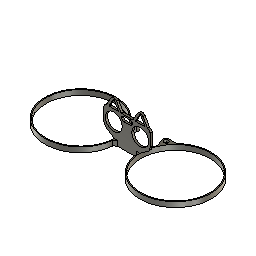
Prop Guard Front v35 (Autodesk Fusion 360 design; units mm, degrees)
Autodesk Fusion 360 part; units mm, degrees
note: some values were not read from the file. Chosen so that the rebuilt part matches the saved one: which face or edge a step refers to; which pieces of a blend or face edit are solid. Set by a fixed rule: which sketch regions a step uses.
sketch "Sketch1" plane through (0, 0, 0) normal (0, 0, 1) x (1, 0, 0)
  line L0 (25, 40) -> (-25, 40)
  line L1 (-25, 40) -> (-25, -40)
  line L2 (-25, -40) -> (25, -40)
  line L3 (25, -40) -> (25, 40)
  line L4 (25, 40) -> (-25, -40) construction
  line L5 (-25, 40) -> (25, -40) construction
  line L6 (25, 40) -> (46.6506, 52.5)
  line L7 (25, 40) -> (55, 40) construction
  line L8 (0, 40) -> (0, -40)
  line L9 (-25, 0) -> (25, 0)
  line L10 (25, 40) -> (23.5, 42.5981)
  line L11 (23.5, 42.5981) -> (45.1506, 55.0981)
  line L12 (45.1506, 55.0981) -> (46.6506, 52.5)
  line L13 (25, 40) -> (26.5, 37.4019)
  line L14 (26.5, 37.4019) -> (48.1506, 49.9019)
  line L15 (23.5, 42.5981) -> (19, 40)
  line L16 (26.5, 37.4019) -> (25, 36.5359)
  line L17 (48.1506, 49.9019) -> (46.6506, 52.5)
  circle A0 centre (46.6506, 52.5) radius 12
  circle A1 centre (46.6506, 52.5) radius 10
  line L18 (46.6506, 52.5) -> (41.6506, 61.1603)
  line L19 (46.6506, 52.5) -> (55.3109, 57.5)
  line L20 (46.6506, 52.5) -> (51.6506, 43.8397)
  circle A2 centre (46.6506, 52.5) radius 1.5
  line L21 (46.6506, 52.5) -> (51.8468, 55.5)
  line L22 (46.6506, 52.5) -> (43.6506, 57.6962)
  circle A3 centre (-46.6506, 52.5) radius 1.5
  line L23 (-23.5, 42.5981) -> (-45.1506, 55.0981)
  line L24 (-26.5, 37.4019) -> (-48.1506, 49.9019)
  circle A4 centre (-46.6506, 52.5) radius 12
  circle A5 centre (-46.6506, 52.5) radius 10
  line L25 (-26.5, 37.4019) -> (-25, 36.5359)
  line L26 (-23.5, 42.5981) -> (-19, 40)
  circle A6 centre (-46.6506, -52.5) radius 10
  line L27 (-26.5, -37.4019) -> (-48.1506, -49.9019)
  line L28 (-23.5, -42.5981) -> (-45.1506, -55.0981)
  line L29 (-23.5, -42.5981) -> (-19, -40)
  line L30 (-26.5, -37.4019) -> (-25, -36.5359)
  line L31 (23.5, -42.5981) -> (19, -40)
  line L32 (26.5, -37.4019) -> (25, -36.5359)
  line L33 (26.5, -37.4019) -> (48.1506, -49.9019)
  line L34 (23.5, -42.5981) -> (45.1506, -55.0981)
  circle A7 centre (46.6506, -52.5) radius 12
  circle A8 centre (46.6506, -52.5) radius 10
  circle A9 centre (46.6506, -52.5) radius 1.5
  circle A10 centre (-46.6506, -52.5) radius 10
  circle A11 centre (-46.6506, -52.5) radius 12
  line L35 (25, 0) -> (25, -40)
  line L36 (0, 0) -> (0, -9)
  line L37 (0, -9) -> (0, -10.6)
  line L38 (0, -9) -> (0, -7.4)
  line L39 (0, -10.6) -> (14, -10.6)
  line L40 (0, -9) -> (1, -9)
  line L41 (0, -7.4) -> (14, -7.4)
  line L42 (14, -10.6) -> (14, -7.4)
  line L43 (-14, -10.6) -> (-14, -7.4)
  line L44 (0, -7.4) -> (-14, -7.4)
  line L45 (0, -10.6) -> (-14, -10.6)
  line L46 (0, 7.4) -> (-14, 7.4)
  line L47 (-14, 10.6) -> (-14, 7.4)
  line L48 (0, 10.6) -> (-14, 10.6)
  line L49 (0, 10.6) -> (14, 10.6)
  line L50 (0, 7.4) -> (14, 7.4)
  line L51 (14, 10.6) -> (14, 7.4)
  line L52 (19, -40) -> (25.9282, -44)
  line L53 (25, -36.5359) -> (25, -31.5359)
  line L54 (19, -40) -> (16, -40)
  line L55 (14.6699, -37.5) -> (34.8771, -37.5) construction
  circle A12 centre (46.6506, -52.5) radius 35
  circle A13 centre (46.6506, -52.5) radius 34
  circle A14 centre (-46.6506, -52.5) radius 35
  circle A15 centre (-46.6506, -52.5) radius 34
  circle A16 centre (-46.6506, 52.5) radius 35
  circle A17 centre (-46.6506, 52.5) radius 34
  circle A18 centre (46.6506, 52.5) radius 35
  circle A19 centre (46.6506, 52.5) radius 34
  line L56 (46.6506, -52.5) -> (46.6506, 52.5)
  line L57 (46.6506, -52.5) -> (-46.6506, -52.5)
  line L58 (46.6506, -52.5) -> (46.6506, -53.5)
  line L59 (-46.6506, -52.5) -> (-46.6506, -53.5)
  line L60 (-46.6506, -53.5) -> (46.6506, -53.5)
  line L61 (46.6506, -52.5) -> (46.6506, -51.5)
  line L62 (-46.6506, -51.5) -> (46.6506, -51.5)
  line L63 (-46.6506, -52.5) -> (-46.6506, -51.5)
  line L64 (-46.6506, 53.5) -> (46.6506, 53.5)
  line L65 (-46.6506, 51.5) -> (46.6506, 51.5)
  line L66 (46.6506, 0) -> (47.1506, 0)
  line L67 (47.1506, 0) -> (47.1506, -17.5036)
  line L68 (47.1506, 0) -> (47.1506, 17.5036)
  line L69 (46.1506, 0) -> (46.1506, 17.5036)
  line L70 (46.1506, 0) -> (46.1506, -17.5036)
  line L71 (-46.1506, 0) -> (-46.1506, 17.5036)
  line L72 (-47.1506, 0) -> (-47.1506, 17.5036)
  line L73 (-47.1506, 0) -> (-47.1506, -17.5036)
  line L74 (-46.1506, 0) -> (-46.1506, -17.5036)
  line L75 (-47.1506, 0) -> (60, 0)
  line L76 (25, -40) -> (25, -30.5)
  line L77 (25, -30.5) -> (15.5, -30.5)
  circle A20 centre (15.5, -30.5) radius 1.3
  circle A21 centre (15.5, -30.5) radius 3.6
  circle A22 centre (-15.5, -30.5) radius 3.6
  circle A23 centre (-15.5, -30.5) radius 1.3
  line L78 (15.5, -30.5) -> (15.5, -29.2)
  circle A24 centre (15.5, -30.5) radius 2.2
  circle A25 centre (-15.5, -30.5) radius 2.2
  point P0 (-46.6506, -52.5)
  dimension "d1" = 50
  dimension "d2" = 80
  dimension "d4" = 25
  dimension "d5" = 30
  dimension "d6" = 3
  dimension "d7" = 25
  dimension "d8" = 24
  dimension "d9" = 20
  dimension "d10" = 3
  dimension "d11" = 6
  dimension "d13" = 6
  dimension "d23" = 9
  dimension "d24" = 1.6
  dimension "d25" = 1.6
  dimension "d26" = 14
  dimension "d51" = 8
  dimension "d76" = 5
  dimension "d77" = 3
  dimension "d88" = 5
  dimension "d130" = 70
  dimension "d131" = 68
  dimension "d132" = 1
  dimension "d133" = 0.5
  dimension "d140" = 9.5
  dimension "d141" = 9.5
  dimension "d142" = 2.6
  dimension "d143" = 7.2
  dimension "d147" = 4.4
  constraint horizontal L0
  constraint perpendicular L0 L1
  constraint parallel L0 L2
  constraint parallel L1 L3
  constraint coincident L4 L36.start
  constraint coincident L5 L36.start
  constraint coincident L36.start origin
  constraint horizontal L7
  constraint midpoint L0 L8.start
  constraint midpoint L2 L8.end
  constraint midpoint L1 L9.start
  constraint midpoint L3 L9.end
  constraint perpendicular L6 L10
  constraint perpendicular L10 L11
  constraint symmetric L0.start L6 L3.end
  constraint symmetric L6 L10.end L13.end
  constraint symmetric L6 L11.end L14.end
  constraint coincident L0 L15.end
  constraint perpendicular L10 L15
  constraint coincident L3 L16.end
  constraint perpendicular L13 L16
  constraint symmetric L12.end L6 L17.end
  constraint coincident L6.end L12.end
  constraint concentric A0 A1
  constraint coincident A1 L18.end
  constraint parallel L12 L18
  constraint coincident A1 L19.end
  constraint perpendicular L12 L19
  constraint coincident A1 L20.end
  constraint perpendicular L19 L20
  constraint perpendicular L20 L21
  constraint parallel L18 L22
  constraint symmetric L8 L10.end L23.start
  constraint symmetric L8 L11.end L23.end
  constraint symmetric L8 L13.end L24.start
  constraint symmetric L8 L14.end L24.end
  constraint symmetric L8 L15.end L26.end
  constraint symmetric L8 L16.end L25.end
  constraint symmetric L8 A0 A4
  constraint symmetric L8 A1 A5
  constraint symmetric L8 A2 A3
  constraint symmetric L9 L10.end L31.start
  constraint symmetric L9 L11.end L34.end
  constraint symmetric L9 L13.end L32.start
  constraint symmetric L9 L14.end L33.end
  constraint symmetric L9 L15.end L31.end
  constraint symmetric L9 L16.end L32.end
  constraint symmetric L9 A0 A7
  constraint symmetric L9 A1 A8
  constraint symmetric L9 A2 A9
  constraint symmetric L9 L23.start L28.start
  constraint symmetric L9 L23.end L28.end
  constraint symmetric L9 L24.start L27.start
  constraint symmetric L9 L24.end L27.end
  constraint symmetric L9 A3.centre P0
  constraint symmetric L9 A5 A6
  constraint symmetric L9 L25.end L30.end
  constraint symmetric L9 L26.end L29.end
  constraint symmetric L9 A5 A10
  constraint symmetric L9 A4 A11
  constraint perpendicular L9 L36
  constraint parallel L8 L37
  constraint parallel L36 L38
  constraint perpendicular L37 L39
  constraint perpendicular L38 L40
  constraint symmetric L37.end L40 L38.end
  constraint symmetric L39.end L40 L41.end
  constraint symmetric L8 L37.end L39.start
  constraint symmetric L8 L39.end L43.start
  constraint symmetric L8 L38.end L41.start
  constraint symmetric L8 L41.end L43.end
  constraint symmetric L9 L37.end L48.start
  constraint symmetric L9 L39.end L49.end
  constraint symmetric L9 L38.end L46.start
  constraint symmetric L9 L41.end L50.end
  constraint symmetric L9 L43.start L47.start
  constraint symmetric L9 L43.end L46.end
  constraint parallel L34 L52
  constraint parallel L2 L54
  constraint horizontal L55
  constraint concentric A8 A12
  constraint concentric A9 A13
  constraint symmetric L8 A12 A14
  constraint symmetric L8 A13 A15
  constraint symmetric L9 A12 A18
  constraint symmetric L9 A13 A19
  constraint symmetric L9 A14 A16
  constraint symmetric L9 A15 A17
  constraint coincident A7.centre A8.centre
  constraint coincident P0 A6.centre
  constraint perpendicular L57 L58
  constraint symmetric L8 A7.centre P0
  constraint symmetric L8 L58.end L59.end
  constraint symmetric L57 A7.centre A8.centre
  constraint symmetric L57 L58.end L61.end
  constraint symmetric L57 P0 A6.centre
  constraint symmetric L57 L59.end L62.start
  constraint symmetric L9 L58.end L64.end
  constraint symmetric L9 L59.end L64.start
  constraint symmetric L9 L61.end L65.end
  constraint symmetric L9 L62.start L65.start
  constraint midpoint L56 L66.start
  constraint perpendicular L56 L66
  constraint coincident A12 L67.end
  constraint perpendicular L66 L67
  constraint coincident A18 L68.end
  constraint perpendicular L66 L68
  constraint symmetric L56 L66.end L69.start
  constraint symmetric L56 L67.end L70.end
  constraint symmetric L56 L68.end L69.end
  constraint symmetric L8 L66.end L72.start
  constraint symmetric L8 L67.end L73.end
  constraint symmetric L8 L68.end L72.end
  constraint symmetric L8 L69.start L71.start
  constraint symmetric L8 L69.end L71.end
  constraint symmetric L8 L70.end L74.end
  constraint perpendicular L71 L75
  constraint perpendicular L2 L76
  constraint perpendicular L35 L77
  constraint coincident L77.end A20.centre
  constraint concentric A20 A21
  constraint symmetric L8 A20 A23
  constraint symmetric L8 A21 A22
  constraint coincident A20 L78.end
  constraint perpendicular L77 L78
  constraint concentric A20 A24
  constraint symmetric L8 A24 A25
  measures "d1" distance of L1.end L2.end
  measures "d2" distance of L0.end L1.end
  measures "d4" distance of L0.start L6.end
  measures "d5" angle of L6 L7
  measures "d6" distance of L0.start L10.end
  measures "d7" distance of L10.end L11.end
  measures "d8" diameter of A0
  measures "d9" diameter of A1
  measures "d10" diameter of A2
  measures "d11" distance of L6.end L21.end
  measures "d13" distance of L6.end L22.end
  measures "d23" distance of L36.start L36.end
  measures "d24" distance of L36.end L37.end
  measures "d25" distance of L36.end L38.end
  measures "d26" distance of L37.end L39.end
  measures "d51" distance of L31.end L52.end
  measures "d76" distance of L32.end L53.end
  measures "d77" distance of L31.end L54.end
  measures "d88" distance of L31.end L55.start
  measures "d130" diameter of A12
  measures "d131" diameter of A13
  measures "d132" distance of A7.centre L58.end
  measures "d133" distance of L66.start L66.end
  measures "d140" distance of L2.end L76.end
  measures "d141" distance of L76.end L77.end
  measures "d142" diameter of A20
  measures "d143" diameter of A21
  measures "d147" diameter of A24
extrude "Extrude6" add sketch "Sketch1" along normal blind 5 contours L3 L35 A12 A13 L56 | L3 L35 A12 A13 L77 | L2 A12 A13 L77 A21 | A12 A13 L56 L60 | A12 A21 | A12 A21 | L1 L2 A14 A15 A22 | L1 A14 A15 L60 | L2 A12 A13 L62 | A14 A22 | A14 A22 | A12 A13 L57 L60 | A12 A13 L57 L62 | L2 A14 A15 L62 | A14 A15 L57 L60 | A12 A14 L57 L60 | A12 A14 L57 L62 | A14 A15 L57 L62 | A24 | A25
chamfer "Chamfer39" distance 5 angle 45 4 edges at (17.1185, -33.7157, 2.5) (19.0718, -30.9499, 2.5) (-19.0718, -30.9499, 2.5) (-17.1185, -33.7157, 2.5)
chamfer "Chamfer40" distance 2 angle 45 4 edges at (11.6649, -51.5, 2.5) (11.6649, -53.5, 2.5) (-11.6649, -51.5, 2.5) (-11.6649, -53.5, 2.5)
extrude "Extrude7" cut sketch "Sketch1" along normal blind 5 and the other way blind -3 contours A24 | A25
sketch "Sketch3" plane through (0, 0, 5) normal (0, 0, 1) x (-1, 0, 0)
  circle A0 centre (-15.5, 30.5) radius 2.2
  circle A1 centre (15.5, 30.5) radius 2.2
  circle A2 centre (46.6506, 52.5) radius 34
  circle A3 centre (-46.6506, 52.5) radius 34
  arc A4 (12.3438, 32.2316) -> (16.0764, 26.9464) centre (15.5, 30.5) ccw
  line L0 (16.0764, 26.9464) -> (22.4239, 27.24)
  arc A5 (22.4239, 27.24) -> (11.7792, 55.4967) centre (46.6506, 52.5) ccw
  line L1 (11.7792, 55.4967) -> (9.6649, 53.5)
  line L2 (9.6649, 53.5) -> (-9.6649, 53.5)
  line L3 (-9.6649, 53.5) -> (-11.7792, 55.4967)
  arc A6 (-11.7792, 55.4967) -> (-22.4239, 27.24) centre (-46.6506, 52.5) ccw
  line L4 (-22.4239, 27.24) -> (-16.0764, 26.9464)
  arc A7 (-16.0764, 26.9464) -> (-12.3438, 32.2316) centre (-15.5, 30.5) ccw
  line L5 (-12.3438, 32.2316) -> (-14.7432, 38.1155)
  arc A8 (-14.7432, 38.1155) -> (-11.7792, 49.5033) centre (-46.6506, 52.5) ccw
  line L6 (-11.7792, 49.5033) -> (-9.6649, 51.5)
  line L7 (-9.6649, 51.5) -> (9.6649, 51.5)
  line L8 (9.6649, 51.5) -> (11.7792, 49.5033)
  arc A9 (11.7792, 49.5033) -> (14.7432, 38.1155) centre (46.6506, 52.5) ccw
  line L9 (14.7432, 38.1155) -> (12.3438, 32.2316)
  line L10 (11.7792, 49.5033) -> (12.783, 49.5033)
  line L11 (11.7792, 55.4967) -> (12.783, 55.4967)
  line L12 (-11.7792, 49.5033) -> (-12.783, 49.5033)
  line L13 (-11.7792, 55.4967) -> (-12.783, 55.4967)
  line L14 (9.6649, 51.5) -> (12.6653, 51.5)
  line L15 (9.6649, 53.5) -> (12.6653, 53.5)
  line L16 (-9.6649, 51.5) -> (-12.6653, 51.5)
  line L17 (-9.6649, 53.5) -> (-12.6653, 53.5)
  line L18 (12.6653, 51.5) -> (22.6653, 51.5)
  line L19 (0, 51.5) -> (0, 53.5)
  line L20 (0, 52.5) -> (12.6506, 52.5)
  line L21 (12.6653, 53.5) -> (22.6653, 53.5)
  line L22 (22.6653, 51.5) -> (22.6653, 53.5)
  line L23 (-12.6653, 51.5) -> (-22.6653, 51.5)
  line L24 (-22.6653, 51.5) -> (-22.6653, 53.5)
  line L25 (-12.6653, 53.5) -> (-22.6653, 53.5)
  dimension "d170" = 10
  constraint coincident L8.end A9.start
  constraint coincident A2 L10.end
  constraint horizontal L10
  constraint coincident A5.end L1.start
  constraint coincident A2 L11.end
  constraint parallel L10 L11
  constraint coincident A8.end L6.start
  constraint coincident A3 L12.end
  constraint parallel L11 L12
  constraint coincident L3.end A6.start
  constraint coincident A3 L13.end
  constraint parallel L7 L13
  constraint coincident L7.end L8.start
  constraint coincident A2 L14.end
  constraint parallel L7 L14
  constraint coincident L1.end L2.start
  constraint coincident A2 L15.end
  constraint parallel L2 L15
  constraint coincident L6.end L7.start
  constraint coincident A3 L16.end
  constraint parallel L7 L16
  constraint coincident L2.end L3.start
  constraint coincident A3 L17.end
  constraint parallel L2 L17
  constraint parallel L14 L18
  constraint midpoint L7 L19.start
  constraint midpoint L2 L19.end
  constraint midpoint L19 L20.start
  constraint coincident A2 L20.end
  constraint perpendicular L19 L20
  constraint symmetric L14.end L20 L15.end
  constraint symmetric L18.end L20 L21.end
  constraint symmetric L14.end L19 L16.end
  constraint symmetric L18.end L19 L23.end
  constraint symmetric L19 L15.end L17.end
  constraint symmetric L19 L21.end L24.end
  measures "d170" distance of L14.end L18.end
extrude "Extrude8" add sketch "Sketch3" along normal blind 35 contours A2 L18 L21 L22 | A2 L2 L15 L19 L20 | A2 L7 L14 L19 L20 | A3 L2 L7 L16 L17 L19 | A3 L23 L24 L25 picked at (19.3271, 52.5) picked at (-19.3271, 52.5)
sketch "Sketch5" plane through (0, -53.5, 0) normal (0, -1, 0) x (1, 0, 0)
  line L0 (-9.6649, 5) -> (-9.6649, 0)
  line L1 (-9.6649, 0) -> (9.6649, 0)
  line L2 (9.6649, 0) -> (9.6649, 5)
  line L3 (9.6649, 5) -> (12.6653, 5)
  line L4 (12.6653, 5) -> (22.6653, 5)
  line L5 (22.6653, 5) -> (22.6653, 40)
  line L6 (22.6653, 40) -> (-22.6653, 40)
  line L7 (-22.6653, 40) -> (-22.6653, 5)
  line L8 (-22.6653, 5) -> (-12.6653, 5)
  line L9 (-12.6653, 5) -> (-9.6649, 5)
  line L10 (0, 40) -> (0, 19)
  line L11 (0, 19) -> (-13, 19)
  circle A0 centre (-13, 19) radius 8.25
  circle A1 centre (13, 19) radius 8.25
  line L12 (0, 40) -> (0, 30)
  line L13 (0, 30) -> (-22.6653, 30)
  line L14 (-22.6653, 30) -> (-12.3126, 30) construction
  line L15 (22.6653, 30) -> (12.3126, 30) construction
  line L16 (0, 30) -> (22.6653, 30)
  line L17 (0, 40) -> (0, 28.5)
  line L18 (0, 28.5) -> (-5.2, 28.5)
  line L19 (-5.2, 28.5) -> (-5.2, 24)
  line L20 (0, 28.5) -> (5.2, 28.5)
  line L21 (5.2, 28.5) -> (5.2, 24)
  line L22 (5.2, 24) -> (-5.2, 24)
  line L23 (-22.6653, 30) -> (-12.0236, 30) construction
  line L24 (0, 19) -> (0, 10.5)
  line L25 (5.4, 12) -> (-5.4, 12)
  line L26 (-5.4, 12) -> (-5.4, 9)
  line L27 (-5.4, 9) -> (5.4, 9)
  line L28 (5.4, 9) -> (5.4, 12)
  line L29 (5.4, 12) -> (-5.4, 9) construction
  line L30 (-5.4, 12) -> (5.4, 9) construction
  line L31 (-13, 19) -> (-13, 40)
  line L32 (-13, 40) -> (-11.5, 40)
  line L33 (-11.5, 40) -> (-5.7265, 30)
  line L34 (-14.5, 40) -> (-20.2735, 30)
  line L35 (11.5, 40) -> (5.7265, 30)
  line L36 (14.5, 40) -> (20.2735, 30)
  line L37 (-13, 40) -> (-13, 38)
  line L38 (-17.3868, 35) -> (-15.6547, 34)
  line L39 (-15.6547, 34) -> (-17.9641, 30)
  line L40 (-13, 38) -> (-15.6547, 38)
  line L41 (-15.6547, 34) -> (-13.3453, 38)
  line L42 (-15.6547, 34) -> (-11.3, 34) construction
  line L43 (-10.3453, 34) -> (-12.6547, 38)
  line L44 (-13, 38) -> (-10.3453, 38)
  line L45 (-10.3453, 34) -> (-8.0359, 30)
  line L46 (10.3453, 34) -> (12.6547, 38)
  line L47 (15.6547, 34) -> (13.3453, 38)
  line L48 (13, 38) -> (10.3453, 38)
  line L49 (13, 38) -> (15.6547, 38)
  line L50 (10.3453, 34) -> (8.0359, 30)
  line L51 (15.6547, 34) -> (17.9641, 30)
  point P0 (0, 10.5)
  dimension "d171" = 21
  dimension "d172" = 13
  dimension "d173" = 16.5
  dimension "d176" = 10
  dimension "d189" = 11.5
  dimension "d190" = 5.2
  dimension "d191" = 4.5
  dimension "d213" = 8.5
  dimension "d230" = 10.8
  dimension "d231" = 3
  dimension "d232" = 1.5
  dimension "d233" = 120
  dimension "d240" = 2
  dimension "d241" = 2
  dimension "d242" = 90
  dimension "d243" = 60
  constraint midpoint L6 L10.start
  constraint perpendicular L6 L10
  constraint perpendicular L10 L11
  constraint coincident L11.end A0.centre
  constraint symmetric L10 A0 A1
  constraint perpendicular L6 L12
  constraint coincident L7 L13.end
  constraint perpendicular L7 L13
  constraint horizontal L14
  constraint symmetric L13.start L12 L16.start
  constraint symmetric L12 L13.end L15.start
  constraint symmetric L12 L14.end L15.end
  constraint perpendicular L6 L17
  constraint perpendicular L12 L18
  constraint perpendicular L18 L19
  constraint symmetric L12 L17.end L18.start
  constraint symmetric L12 L18.end L20.end
  constraint symmetric L12 L19.end L21.end
  constraint horizontal L23
  constraint perpendicular L11 L24
  constraint horizontal L25
  constraint perpendicular L25 L26
  constraint parallel L25 L27
  constraint parallel L26 L28
  constraint coincident L29 P0
  constraint coincident L30 P0
  constraint coincident P0 L24.end
  constraint coincident L6 L31.end
  constraint perpendicular L6 L31
  constraint perpendicular L31 L32
  constraint coincident L13 L33.end
  constraint symmetric L31 L32.end L34.start
  constraint symmetric L31 L33.end L34.end
  constraint symmetric L17 L32.end L35.start
  constraint symmetric L17 L33.end L35.end
  constraint symmetric L17 L34.start L36.start
  constraint symmetric L17 L34.end L36.end
  constraint coincident L31 L37.end
  constraint midpoint L34 L38.start
  constraint perpendicular L34 L38
  constraint coincident L14 L39.end
  constraint coincident L34 L40.end
  constraint perpendicular L37 L40
  constraint horizontal L42
  constraint coincident L40 L41.end
  constraint symmetric L31 L37.end L40.start
  constraint symmetric L31 L38.end L43.start
  constraint symmetric L31 L39.end L45.end
  constraint symmetric L31 L40.end L44.end
  constraint symmetric L31 L41.end L43.end
  constraint symmetric L12 L37.end L48.start
  constraint symmetric L12 L38.end L47.start
  constraint symmetric L12 L39.end L51.end
  constraint symmetric L12 L40.end L49.end
  constraint symmetric L12 L41.end L47.end
  constraint symmetric L12 L43.start L46.start
  constraint symmetric L12 L43.end L46.end
  constraint symmetric L12 L44.end L48.end
  constraint symmetric L12 L45.end L50.end
  measures "d171" distance of L10.start L10.end
  measures "d172" distance of L10.end L11.end
  measures "d173" diameter of A0
  measures "d176" distance of L10.start L12.end
  measures "d189" distance of L10.start L17.end
  measures "d190" distance of L17.end L18.end
  measures "d191" distance of L18.end L19.end
  measures "d213" distance of L10.end P0
  measures "d230" distance of L26.end L27.end
  measures "d231" distance of L25.end L26.end
  measures "d232" distance of L31.end L32.end
  measures "d233" angle of L32 L33
  measures "d240" distance of L31.end L37.end
  measures "d241" distance of L38.start L38.end
  measures "d242" angle of L38 L39
  measures "d243" angle of L41 L42
extrude "Extrude12" cut sketch "Sketch5" against normal blind 2 contours L6 L7 L13 L34 | L13 L31 L39 L40 L41 | L5 L6 L16 L36 | L13 L31 L43 L44 L45 | L6 L10 L12 L13 L17 L33 | L11 A0 L31 | L11 A0 L31 | L16 L46 L47 L48 L49 L50 L51 | L6 L10 L12 L16 L17 L35 | L10 L20 L21 L22 | L10 L18 L19 L22 | A1
fillet "Fillet7" radius 2 4 edges at (5.2, -52.5, 28.5) (5.2, -52.5, 24) (-5.2, -52.5, 24) (-5.2, -52.5, 28.5)
chamfer "Chamfer41" distance 7 distance2 10 1 edges at (-22.6653, -52.5, 5) measured on face at (-22.6653, -52.1667, 13.3333)
chamfer "Chamfer42" distance 10 distance2 7 1 edges at (22.6653, -52.5, 5) measured on face at (19.3277, -52.3889, 5)
fillet "Fillet17" radius 3.25 4 edges at (-11.5, -52.5, 40) (-14.5, -52.5, 40) (14.5, -52.5, 40) (11.5, -52.5, 40)
fillet "Fillet18" radius 0.5 8 edges at (-12.6547, -52.5, 38) (-13.3453, -52.5, 38) (13.3453, -52.5, 38) (12.6547, -52.5, 38) (17.9641, -52.5, 30) (-8.0359, -52.5, 30) (8.0359, -52.5, 30) (-17.9641, -52.5, 30)
fillet "Fillet19" radius 5.25 2 edges at (-22.6653, -52.5, 12) (22.6653, -52.5, 12)
fillet "Fillet21" radius 3 2 edges at (-22.6653, -52.5, 30) (22.6653, -52.5, 30)
extrude "Extrude13" cut sketch "Sketch5" along normal blind -2 and the other way blind 1 contours L25 L26 L27 L28
chamfer "Chamfer45" distance 2 angle 45 2 edges at (-11.1651, -51.5, 5) (11.1651, -51.5, 5)
equation "d143 = 3.2 mm + 4 mm"
